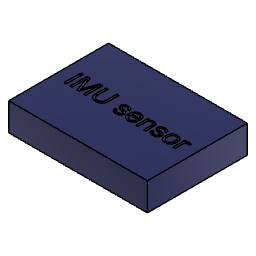
IMU sensor v1 (Autodesk Fusion 360 design; units mm, degrees)
Autodesk Fusion 360 part; units mm, degrees
sketch "Sketch1" plane through (0, 0, 0) normal (0, 0, 1) x (1, 0, 0)
  line L0 (0, 0) -> (25, 0)
  line L1 (25, 0) -> (25, 18)
  line L2 (25, 18) -> (0, 18)
  line L3 (0, 18) -> (0, 0)
  dimension "d1" = 25
  dimension "d2" = 18
  constraint horizontal L0
  constraint vertical L1
  constraint horizontal L2
  constraint vertical L3
  constraint coincident L0.start L3.end
  measures "d1" distance of L0.start L0.end
  measures "d2" distance of L0.start L2.end
extrude "Extrude1" add sketch "Sketch1" along normal blind 5
sketch "Sketch2" plane through (0, 0, 5) normal (0, 0, 1) x (-1, 0, 0)
  line L0 (0, -18) -> (0, 0)
  line L1 (0, 0) -> (-25, 0)
  line L2 (-25, 0) -> (-25, -18)
  line L3 (-25, -18) -> (0, -18)
  line L4 (-2.096, -5.6815) -> (-24.9212, -5.335) construction
  line L5 (-24.9212, -5.335) -> (-25, -10.5236) construction
  line L6 (-25, -10.5236) -> (-2.1747, -10.87) construction
  line L7 (-2.1747, -10.87) -> (-2.096, -5.6815) construction
  dimension "d5" = 3
  text T0 "IMU sensor" font "Arial" height 3 align left top in box 22.8279 x 5.1892 at (-2.096, -5.6815) x (-0.999885, 0.015176) y (-0.015176, -0.999885) spacing 1
  constraint coincident L2
extrude "Extrude2" cut sketch "Sketch2" against normal blind 1 text T0
